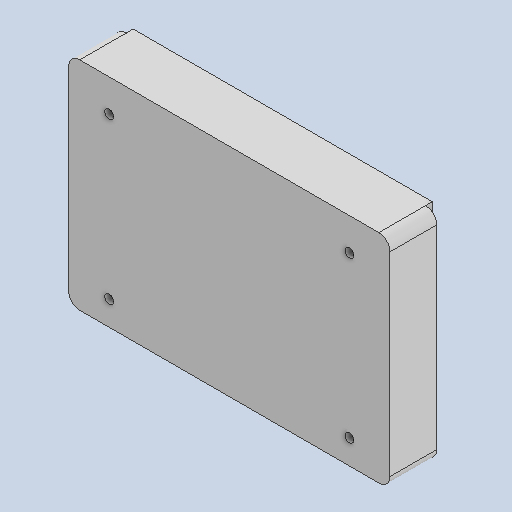
# Autodesk Inventor part: ThermalConductivityBlock_NX
Saved by Autodesk Inventor 2024.2 (Build 282272000, 272)
## iProperties
Created: 2020-06-17
Part Number: ThermalConductivityBlock_NX
Material: Generic
Document SubType Name: Modeling
Designer: Viktor Lindström
Density: 1 g/cm^3
Appearance: Default
Author: Viktor Lindström
Autodesk Inventor part; units mm, degrees
ref_plane "YZ Plane" through (0, 0, 0) normal (1, 0, 0) x (0, 1, 0)
ref_plane "XZ Plane" through (0, 0, 0) normal (0, 1, 0) x (-1, 0, 0)
ref_plane "XY Plane" through (0, 0, 0) normal (0, 0, 1) x (1, 0, 0)
sketch "Sketch1" plane through (0, 0, 0) normal (0, 0, 1) x (1, 0, 0)
  line L0 (-28.9, -19.5) -> (28.9, -19.5)
  line L1 (28.9, -19.5) -> (28.9, 19.5)
  line L2 (28.9, 19.5) -> (-28.9, 19.5)
  line L3 (-28.9, 19.5) -> (-28.9, -19.5)
  line L4 (-28.9, -19.5) -> (28.9, 19.5) construction
  line L5 (28.9, -19.5) -> (-28.9, 19.5) construction
  point P0 (0, 0)
  dimension "d0" = 57.8
  dimension "d1" = 39
  constraints: 12 end point, 2 midpoint, 2 parallel, 1 horizontal, 1 perpendicular
  measures "d0" distance of L1.end L2.end
  measures "d1" distance of L2.end L0.start
extrude "Extrusion1" add sketch "Sketch1" along normal blind 9.61
sketch "Sketch2" plane through (0, 0, 0) normal (0, 0, -1) x (-1, 0, 0)
  circle A0 centre (-21.6, -15.1) radius 0.8
  line L0 (55.7735, 0) -> (-51.4211, 0) construction
  line L1 (0, -27.3) -> (0, 27.3) construction
  line L2 (28.9, -19.5) -> (-28.9, -19.5) projected
  line L3 (-28.9, -19.5) -> (-28.9, 19.5) projected
  circle A1 centre (21.6, -15.1) radius 0.8
  line L4 (-36.1076, -0.7) -> (40.46, -0.7) construction
  circle A2 centre (-21.6, 13.7) radius 0.8
  circle A3 centre (21.6, 13.7) radius 0.8
  line L5 (-28.9, 19.5) -> (28.9, 19.5) projected
  point P0 (0, 0)
  dimension "d4" = 1.6
  dimension "d5" = 4.4
  dimension "d6" = 7.3
  dimension "d7" = 5.8
  constraints: 4 centre point, 3 symmetric about line, 2 end point, 1 horizontal, 3 other
  measures "d4" diameter of A0
  measures "d5" distance from line of L2 A0.centre
  measures "d6" distance from line of L3 A0.centre
  measures "d7" distance from line of L5 A2.centre
extrude "Extrusion2" cut sketch "Sketch2" against normal through all
sketch "Sketch3" plane through (0, 0, 0) normal (0, 0, -1) x (-1, 0, 0)
  line L0 (-28.9, 19.5) -> (28.9, 19.5) construction
  line L1 (28.9, -19.5) -> (-28.9, -19.5) construction
  line L2 (-28.9, -19.5) -> (-28.9, 19.5) projected
  line L3 (-26.9, 19.5) -> (-26.9, -0.4)
  line L4 (-24.9, -2.4) -> (-19.85, -2.4)
  line L5 (-17.85, -4.4) -> (-17.85, -11.3)
  line L6 (-19.85, -13.3) -> (-24.9, -13.3)
  line L7 (-26.9, -15.3) -> (-26.9, -19.5)
  line L8 (-28.9, 19.5) -> (28.9, 19.5) projected
  line L9 (-26.9, 19.5) -> (-28.9, 19.5)
  line L10 (-28.9, 19.5) -> (-28.9, -19.5)
  arc A0 (-26.9, -0.4) -> (-24.9, -2.4) centre (-24.9, -0.4) ccw
  arc A1 (-17.85, -4.4) -> (-19.85, -2.4) centre (-19.85, -4.4) ccw
  arc A2 (-19.85, -13.3) -> (-17.85, -11.3) centre (-19.85, -11.3) ccw
  arc A3 (-24.9, -13.3) -> (-26.9, -15.3) centre (-24.9, -15.3) ccw
  line L11 (-28.9, 19.5) -> (-26.9, 19.5)
  line L12 (-28.9, -19.5) -> (-28.9, 19.5) projected
  line L13 (-28.9, -19.5) -> (-26.9, -19.5)
  line L14 (0, -27.3) -> (0, 27.3) projected
  line L15 (28.9, -19.5) -> (28.9, 19.5)
  line L16 (26.9, 19.5) -> (26.9, -0.4)
  line L17 (24.9, -2.4) -> (19.85, -2.4)
  line L18 (17.85, -4.4) -> (17.85, -11.3)
  line L19 (19.85, -13.3) -> (24.9, -13.3)
  line L20 (26.9, -15.3) -> (26.9, -19.5)
  line L21 (26.9, 19.5) -> (28.9, 19.5)
  line L22 (28.9, 19.5) -> (28.9, -19.5)
  arc A4 (24.9, -2.4) -> (26.9, -0.4) centre (24.9, -0.4) ccw
  arc A5 (19.85, -2.4) -> (17.85, -4.4) centre (19.85, -4.4) ccw
  arc A6 (17.85, -11.3) -> (19.85, -13.3) centre (19.85, -11.3) ccw
  arc A7 (26.9, -15.3) -> (24.9, -13.3) centre (24.9, -15.3) ccw
  line L23 (28.9, 19.5) -> (26.9, 19.5)
  line L24 (28.9, -19.5) -> (28.9, 19.5)
  line L25 (28.9, -19.5) -> (26.9, -19.5)
  point P0 (0, 0)
  point P1 (-26.9, -13.3)
  point P2 (26.9, -13.3)
  dimension "d10" = 6.2
  dimension "d11" = 21.9
  dimension "d12" = 11.05
  dimension "d13" = 2
  dimension "d14" = 2
  constraints: 40 end point, 16 point on circle, 15 symmetric about line, 10 point on line, 8 centre point, 8 tangent, 5 perpendicular, 3 equal radius, 1 collinear, 1 parallel, 1 vertical, 4 other
  measures "d10" distance between parallel lines of L1 L6
  measures "d11" distance between parallel lines of L0 L4
  measures "d12" distance between parallel lines of L5 L2
  measures "d13" distance between parallel lines of L2 L3
  measures "d14" radius of A0
extrude "Extrusion3" cut sketch "Sketch3" against normal blind 1.2
fillet "Fillet1" radius 2 4 edges at (-28.9, 19.5, 5.405) (28.9, 19.5, 5.405) (28.9, -19.5, 5.405) (-28.9, -19.5, 5.405)
body "Solid1"
